Autodesk Inventor part; units mm, degrees
(part 2 of 7)
  arc A582 (128.3559, 101.1967) -> (128.4338, 100.8049) centre (148.5, 105) ccw
  arc A583 (128.7164, 99.628) -> (128.8248, 99.2435) centre (148.5, 105) ccw
  arc A584 (129.1989, 98.0923) -> (129.3371, 97.7175) centre (148.5, 105) ccw
  arc A585 (129.8003, 96.5993) -> (129.9676, 96.2365) centre (148.5, 105) ccw
  arc A586 (130.5171, 95.158) -> (130.7123, 94.8095) centre (148.5, 105) ccw
  arc A587 (131.3447, 93.7774) -> (131.5666, 93.4453) centre (148.5, 105) ccw
  arc A588 (132.2781, 92.466) -> (132.5254, 92.1523) centre (148.5, 105) ccw
  arc A589 (133.3115, 91.2319) -> (133.5827, 90.9386) centre (148.5, 105) ccw
  arc A590 (134.4386, 90.0827) -> (134.7319, 89.8115) centre (148.5, 105) ccw
  arc A591 (135.6523, 89.0254) -> (135.966, 88.7781) centre (148.5, 105) ccw
  arc A592 (136.9453, 88.0666) -> (137.2774, 87.8447) centre (148.5, 105) ccw
  arc A593 (138.3095, 87.2123) -> (138.658, 87.0171) centre (148.5, 105) ccw
  arc A594 (139.7365, 86.4676) -> (140.0993, 86.3003) centre (148.5, 105) ccw
  arc A595 (141.2175, 85.8371) -> (141.5923, 85.6989) centre (148.5, 105) ccw
  arc A596 (142.7435, 85.3248) -> (143.128, 85.2164) centre (148.5, 105) ccw
  arc A597 (144.3049, 84.9338) -> (144.6967, 84.8559) centre (148.5, 105) ccw
  arc A598 (145.8922, 84.6665) -> (146.2889, 84.6196) centre (148.5, 105) ccw
  arc A599 (147.4956, 84.5246) -> (147.8948, 84.5089) centre (148.5, 105) ccw
  arc A600 (149.1052, 84.5089) -> (149.5044, 84.5246) centre (148.5, 105) ccw
  arc A601 (150.7111, 84.6196) -> (151.1078, 84.6665) centre (148.5, 105) ccw
  arc A602 (152.3033, 84.8559) -> (152.6951, 84.9338) centre (148.5, 105) ccw
  arc A603 (153.872, 85.2164) -> (154.2565, 85.3248) centre (148.5, 105) ccw
  arc A604 (155.4077, 85.6989) -> (155.7825, 85.8371) centre (148.5, 105) ccw
  arc A605 (156.9007, 86.3003) -> (157.2635, 86.4676) centre (148.5, 105) ccw
  arc A606 (158.342, 87.0171) -> (158.6905, 87.2123) centre (148.5, 105) ccw
  arc A607 (159.7226, 87.8447) -> (160.0547, 88.0666) centre (148.5, 105) ccw
  arc A608 (161.034, 88.7781) -> (161.3477, 89.0254) centre (148.5, 105) ccw
  arc A609 (162.2681, 89.8115) -> (162.5614, 90.0827) centre (148.5, 105) ccw
  arc A610 (163.4173, 90.9386) -> (163.6885, 91.2319) centre (148.5, 105) ccw
  arc A611 (164.4746, 92.1523) -> (164.7219, 92.466) centre (148.5, 105) ccw
  arc A612 (165.4334, 93.4453) -> (165.6553, 93.7774) centre (148.5, 105) ccw
  arc A613 (166.2877, 94.8095) -> (166.4829, 95.158) centre (148.5, 105) ccw
  arc A614 (167.0324, 96.2365) -> (167.1997, 96.5993) centre (148.5, 105) ccw
  arc A615 (167.6629, 97.7175) -> (167.8011, 98.0923) centre (148.5, 105) ccw
  arc A616 (168.1752, 99.2435) -> (168.2836, 99.628) centre (148.5, 105) ccw
  arc A617 (168.5662, 100.8049) -> (168.6441, 101.1967) centre (148.5, 105) ccw
  arc A618 (168.8335, 102.3922) -> (168.8804, 102.7889) centre (148.5, 105) ccw
  arc A619 (168.9754, 103.9956) -> (168.9911, 104.3948) centre (148.5, 105) ccw
  arc A620 (168.9911, 105.6052) -> (168.9754, 106.0044) centre (148.5, 105) ccw
  arc A621 (168.8804, 107.2111) -> (168.8335, 107.6078) centre (148.5, 105) ccw
  arc A622 (168.6441, 108.8033) -> (168.5662, 109.1951) centre (148.5, 105) ccw
  arc A623 (168.2836, 110.372) -> (168.1752, 110.7565) centre (148.5, 105) ccw
  arc A624 (167.8011, 111.9077) -> (167.6629, 112.2825) centre (148.5, 105) ccw
  arc A625 (167.1997, 113.4007) -> (167.0324, 113.7635) centre (148.5, 105) ccw
  arc A626 (166.4829, 114.842) -> (166.2877, 115.1905) centre (148.5, 105) ccw
  arc A627 (165.6553, 116.2226) -> (165.4334, 116.5547) centre (148.5, 105) ccw
  arc A628 (164.7219, 117.534) -> (164.4746, 117.8477) centre (148.5, 105) ccw
  arc A629 (163.6885, 118.7681) -> (163.4173, 119.0614) centre (148.5, 105) ccw
  arc A630 (162.5614, 119.9173) -> (162.2681, 120.1885) centre (148.5, 105) ccw
  arc A631 (161.3477, 120.9746) -> (161.034, 121.2219) centre (148.5, 105) ccw
  arc A632 (160.0547, 121.9334) -> (159.7226, 122.1553) centre (148.5, 105) ccw
  arc A633 (158.6905, 122.7877) -> (158.342, 122.9829) centre (148.5, 105) ccw
  arc A634 (157.2635, 123.5324) -> (156.9007, 123.6997) centre (148.5, 105) ccw
  arc A635 (155.7825, 124.1629) -> (155.4077, 124.3011) centre (148.5, 105) ccw
  arc A636 (154.2565, 124.6752) -> (153.872, 124.7836) centre (148.5, 105) ccw
  arc A637 (152.6951, 125.0662) -> (152.3033, 125.1441) centre (148.5, 105) ccw
  arc A638 (151.1078, 125.3335) -> (150.7111, 125.3804) centre (148.5, 105) ccw
  arc A639 (149.5044, 125.4754) -> (149.1052, 125.4911) centre (148.5, 105) ccw
  line L0 (126, 105) -> (171, 105)
  line L1 (148.5, 82.5) -> (148.5, 127.5)
  line L2 (189, 125.5) -> (259, 125.5)
  line L3 (189, 117.5) -> (259, 117.5)
  line L4 (189, 109.5) -> (259, 109.5)
  line L5 (189, 101.5) -> (259, 101.5)
  line L6 (189, 93.5) -> (259, 93.5)
  line L7 (189, 85.5) -> (259, 85.5)
  line L8 (189, 77.5) -> (259, 77.5)
  line L9 (189, 69.5) -> (259, 69.5)
  line L10 (189, 61.5) -> (259, 61.5)
  line L11 (189, 53.5) -> (259, 53.5)
  line L12 (189, 45.5) -> (259, 45.5)
  line L13 (189, 37.5) -> (259, 37.5)
  line L14 (189, 29.5) -> (259, 29.5)
  line L15 (189, 125.5) -> (189, 29.5)
  line L16 (259, 125.5) -> (259, 29.5)
  line L17 (224, 117.5) -> (224, 29.5)
  arc A640 (149.1982, 109.7586) -> (149.1615, 109.6213) centre (149.7545, 109.5365) ccw
  arc A641 (149.402, 110.1264) -> (149.1982, 109.7586) centre (150.7515, 109.1382) ccw
  arc A642 (150.0725, 110.7903) -> (149.402, 110.1264) centre (151.8157, 108.3591) ccw
  arc A643 (146.2672, 109.2599) -> (146.3182, 109.1272) centre (146.8478, 109.4071) ccw
  arc A644 (146.2159, 109.6791) -> (146.2672, 109.2599) centre (147.8885, 109.671) ccw
  arc A645 (146.3688, 110.6087) -> (146.2159, 109.6791) centre (149.2074, 109.6645) ccw
  arc A646 (144.1897, 107.1339) -> (144.309, 107.0566) centre (144.5729, 107.5943) ccw
  arc A647 (143.9018, 107.4429) -> (144.1897, 107.1339) centre (145.2598, 108.4195) ccw
  arc A648 (143.4791, 108.2848) -> (143.9018, 107.4429) centre (146.3305, 109.1895) ccw
  arc A649 (143.7586, 104.1928) -> (143.9006, 104.2004) centre (143.7981, 104.7905) ccw
  arc A650 (143.3441, 104.2736) -> (143.7586, 104.1928) centre (143.8687, 105.8619) ccw
  arc A651 (142.5072, 104.7063) -> (143.3441, 104.2736) centre (144.2823, 107.1142) ccw
  arc A652 (145.1386, 101.5601) -> (145.249, 101.6496) centre (144.8192, 102.0668) ccw
  arc A653 (144.7558, 101.3818) -> (145.1386, 101.5601) centre (144.2466, 102.9751) ccw
  arc A654 (143.8244, 101.2399) -> (144.7558, 101.3818) centre (143.8452, 104.2313) ccw
  arc A655 (147.8018, 100.2415) -> (147.8385, 100.3788) centre (147.2456, 100.4636) ccw
  arc A656 (147.5969, 99.8722) -> (147.8018, 100.2415) centre (146.2485, 100.8619) ccw
  arc A657 (146.9268, 99.2099) -> (147.5969, 99.8722) centre (145.1853, 101.6423) ccw
  arc A658 (150.7315, 100.7396) -> (150.6805, 100.8723) centre (150.1509, 100.5924) ccw
  arc A659 (150.7828, 100.3204) -> (150.7315, 100.7396) centre (149.1102, 100.3285) ccw
  arc A660 (150.6299, 99.3908) -> (150.7828, 100.3204) centre (147.7913, 100.335) ccw
  arc A661 (152.8095, 102.8649) -> (152.6903, 102.9423) centre (152.4263, 102.4046) ccw
  arc A662 (153.0974, 102.5559) -> (152.8095, 102.8649) centre (151.7394, 101.5794) ccw
  arc A663 (153.5202, 101.714) -> (153.0974, 102.5559) centre (150.6687, 100.8093) ccw
  arc A664 (153.2414, 105.8058) -> (153.0995, 105.7982) centre (153.202, 105.2081) ccw
  arc A665 (153.656, 105.725) -> (153.2414, 105.8058) centre (153.1314, 104.1367) ccw
  arc A666 (154.4929, 105.2923) -> (153.656, 105.725) centre (152.7177, 102.8844) ccw
  arc A667 (151.8623, 108.4388) -> (151.7519, 108.3493) centre (152.1817, 107.9321) ccw
  arc A668 (152.2451, 108.6171) -> (151.8623, 108.4388) centre (152.7543, 107.0239) ccw
  arc A669 (153.1765, 108.759) -> (152.2451, 108.6171) centre (153.1557, 105.7676) ccw
  arc A670 (147.8392, 109.6213) -> (147.8025, 109.7587) centre (147.2462, 109.5365) ccw
  arc A671 (147.8025, 109.7587) -> (147.5976, 110.128) centre (146.2492, 109.1383) ccw
  arc A672 (147.5976, 110.128) -> (146.9275, 110.7903) centre (145.186, 108.3579) ccw
  arc A673 (145.2491, 108.3503) -> (145.1386, 108.4399) centre (144.8192, 107.9332) ccw
  arc A674 (145.1386, 108.4399) -> (144.7558, 108.6182) centre (144.2466, 107.0249) ccw
  arc A675 (144.7558, 108.6182) -> (143.8244, 108.7601) centre (143.8452, 105.7687) ccw
  arc A676 (143.9007, 105.7996) -> (143.7586, 105.8072) centre (143.7981, 105.2095) ccw
  arc A677 (143.7586, 105.8072) -> (143.3441, 105.7264) centre (143.8687, 104.1381) ccw
  arc A678 (143.3441, 105.7264) -> (142.5072, 105.2937) centre (144.2823, 102.8858) ccw
  arc A679 (144.309, 102.9435) -> (144.1897, 102.8661) centre (144.5729, 102.4057) ccw
  arc A680 (144.1897, 102.8661) -> (143.9018, 102.5571) centre (145.2598, 101.5805) ccw
  arc A681 (143.9018, 102.5571) -> (143.4791, 101.7152) centre (146.3305, 100.8105) ccw
  arc A682 (146.3189, 100.8726) -> (146.2679, 100.7399) centre (146.8485, 100.5927) ccw
  arc A683 (146.2679, 100.7399) -> (146.2166, 100.3207) centre (147.8892, 100.3288) ccw
  arc A684 (146.2166, 100.3207) -> (146.3695, 99.391) centre (149.2081, 100.3352) ccw
  arc A685 (149.1608, 100.3787) -> (149.1975, 100.2413) centre (149.7538, 100.4635) ccw
  arc A686 (149.1975, 100.2413) -> (149.4024, 99.872) centre (150.7508, 100.8617) ccw
  arc A687 (149.4024, 99.872) -> (150.0725, 99.2097) centre (151.814, 101.6421) ccw
  arc A688 (151.7509, 101.6497) -> (151.8614, 101.5601) centre (152.1808, 102.0668) ccw
  arc A689 (151.8614, 101.5601) -> (152.2442, 101.3818) centre (152.7534, 102.9751) ccw
  arc A690 (152.2442, 101.3818) -> (153.1756, 101.2399) centre (153.1548, 104.2313) ccw
  arc A691 (153.0993, 104.2004) -> (153.2414, 104.1928) centre (153.2019, 104.7905) ccw
  arc A692 (153.2414, 104.1928) -> (153.6559, 104.2736) centre (153.1313, 105.8619) ccw
  arc A693 (153.6559, 104.2736) -> (154.4928, 104.7063) centre (152.7177, 107.1142) ccw
  arc A694 (152.691, 107.0565) -> (152.8103, 107.1339) centre (152.4271, 107.5943) ccw
  arc A695 (152.8103, 107.1339) -> (153.0982, 107.4429) centre (151.7402, 108.4195) ccw
  arc A696 (153.0982, 107.4429) -> (153.5209, 108.2848) centre (150.6695, 109.1895) ccw
  arc A697 (150.6818, 109.1272) -> (150.7328, 109.2599) centre (150.1522, 109.4071) ccw
  arc A698 (150.7328, 109.2599) -> (150.7841, 109.6791) centre (149.1115, 109.671) ccw
  arc A699 (150.7841, 109.6791) -> (150.6312, 110.6087) centre (147.7926, 109.6645) ccw
  arc A700 (149.0314, 108.7125) -> (147.9691, 108.7126) centre (148.5, 105) ccw
  arc A701 (146.7471, 108.3155) -> (145.8883, 107.6915) centre (148.5, 105) ccw
  arc A702 (145.1331, 106.652) -> (144.8051, 105.6424) centre (148.5, 105) ccw
  arc A703 (144.8051, 104.3575) -> (145.1332, 103.3479) centre (148.5, 105) ccw
  arc A704 (145.8884, 102.3084) -> (146.7478, 101.6841) centre (148.5, 105) ccw
  arc A705 (147.9686, 101.2875) -> (149.0308, 101.2874) centre (148.5, 105) ccw
  arc A706 (150.2516, 101.6838) -> (151.1117, 102.3085) centre (148.5, 105) ccw
  arc A707 (151.8663, 103.3467) -> (152.1949, 104.3576) centre (148.5, 105) ccw
  arc A708 (152.1951, 105.6411) -> (151.8668, 106.6521) centre (148.5, 105) ccw
  arc A709 (151.1126, 107.6906) -> (150.2528, 108.3155) centre (148.5, 105) ccw
  arc A710 (146.9275, 110.7903) -> (146.3688, 110.6087) centre (148.5, 105) ccw
  arc A711 (143.8244, 108.7601) -> (143.4791, 108.2848) centre (148.5, 105) ccw
  arc A712 (142.5072, 105.2937) -> (142.5072, 104.7063) centre (148.5, 105) ccw
  arc A713 (143.4791, 101.7152) -> (143.8244, 101.2399) centre (148.5, 105) ccw
  arc A714 (146.3695, 99.391) -> (146.9268, 99.2099) centre (148.5, 105) ccw
  arc A715 (150.0725, 99.2097) -> (150.6299, 99.3908) centre (148.5, 105) ccw
  arc A716 (153.1756, 101.2399) -> (153.5202, 101.714) centre (148.5, 105) ccw
  arc A717 (154.4928, 104.7063) -> (154.4929, 105.2923) centre (148.5, 105) ccw
  arc A718 (153.5209, 108.2848) -> (153.1765, 108.759) centre (148.5, 105) ccw
  arc A719 (150.6312, 110.6087) -> (150.0725, 110.7903) centre (148.5, 105) ccw
  line L18 (149.0314, 108.7125) -> (149.1615, 109.6213)
  line L19 (146.7471, 108.3155) -> (146.3182, 109.1272)
  line L20 (145.1331, 106.652) -> (144.309, 107.0566)
  line L21 (144.8051, 104.3575) -> (143.9006, 104.2004)
  line L22 (145.8884, 102.3084) -> (145.249, 101.6496)
  line L23 (147.9686, 101.2875) -> (147.8385, 100.3788)
  line L24 (150.2516, 101.6838) -> (150.6805, 100.8723)
  line L25 (151.8663, 103.3467) -> (152.6903, 102.9423)
  line L26 (152.1951, 105.6411) -> (153.0995, 105.7982)
  line L27 (151.1126, 107.6906) -> (151.7519, 108.3493)
  line L28 (147.9691, 108.7126) -> (147.8392, 109.6213)
  line L29 (145.8883, 107.6915) -> (145.2491, 108.3503)
  line L30 (144.8051, 105.6424) -> (143.9007, 105.7996)
  line L31 (145.1332, 103.3479) -> (144.309, 102.9435)
  line L32 (146.7478, 101.6841) -> (146.3189, 100.8726)
  line L33 (149.0308, 101.2874) -> (149.1608, 100.3787)
  line L34 (151.1117, 102.3085) -> (151.7509, 101.6497)
  line L35 (152.1949, 104.3576) -> (153.0993, 104.2004)
  line L36 (151.8668, 106.6521) -> (152.691, 107.0565)
  line L37 (150.2528, 108.3155) -> (150.6818, 109.1272)
  line L38 (140.5, 105) -> (156.5, 105)
  line L39 (148.5, 97) -> (148.5, 113)
  line L40 (174.5, 111) -> (244.5, 111)
  line L41 (174.5, 103) -> (244.5, 103)
  line L42 (174.5, 95) -> (244.5, 95)
  line L43 (174.5, 87) -> (244.5, 87)
  line L44 (174.5, 79) -> (244.5, 79)
  line L45 (174.5, 71) -> (244.5, 71)
  line L46 (174.5, 63) -> (244.5, 63)
  line L47 (174.5, 55) -> (244.5, 55)
  line L48 (174.5, 47) -> (244.5, 47)
  line L49 (174.5, 39) -> (244.5, 39)
  line L50 (174.5, 31) -> (244.5, 31)
  line L51 (174.5, 23) -> (244.5, 23)
  line L52 (174.5, 15) -> (244.5, 15)
  line L53 (174.5, 111) -> (174.5, 15)
  line L54 (244.5, 111) -> (244.5, 15)
  line L55 (209.5, 103) -> (209.5, 15)
  point P0 (0, 0)
  point P1 (195, 119.5)
  point P2 (197.5, 111.5)
  point P3 (197.5, 103.5)
  point P4 (195, 95.5)
  point P5 (197.5, 87.5)
  point P6 (192.5, 79.5)
  point P7 (195, 71.5)
  point P8 (195, 63.5)
  point P9 (195, 55.5)
  point P10 (197.5, 47.5)
  point P11 (197.5, 39.5)
  point P12 (195, 31.5)
  point P13 (225, 111.5)
  point P14 (240, 103.5)
  point P15 (238.75, 95.5)
  point P16 (237.5, 87.5)
  point P17 (240, 79.5)
  point P18 (233.75, 71.5)
  point P19 (240, 63.5)
  point P20 (236.25, 55.5)
  point P21 (235, 47.5)
  point P22 (242.5, 39.5)
  point P23 (242.5, 31.5)
  point P24 (149.5, 141)
  point P25 (149.5, 135)
  point P26 (165.6875, 141)
  point P27 (167.8125, 135)
  point P28 (180.5, 105)
  point P29 (183, 97)
  point P30 (183, 89)
  point P31 (180.5, 81)
  point P32 (183, 73)
  point P33 (178, 65)
  point P34 (180.5, 57)
  point P35 (180.5, 49)
  point P36 (180.5, 41)
  point P37 (183, 33)
  point P38 (183, 25)
  point P39 (180.5, 17)
  point P40 (210.5, 97)
  point P41 (225.5, 89)
  point P42 (226.75, 81)
  point P43 (223, 73)
  point P44 (225.5, 65)
  point P45 (220.5, 57)
  point P46 (225.5, 49)
  point P47 (224.25, 41)
  point P48 (220.5, 33)
  point P49 (228, 25)
  point P50 (228, 17)
  point P51 (149.5, 126.5)
  point P52 (149.5, 120.5)
  point P53 (167.8125, 126.5)
  point P54 (168.875, 120.5)
  constraints: 1120 point on circle, 560 centre point, 534 equal radius, 410 tangent, 104 end point, 84 horizontal, 26 parallel, 9 concentric, 4 midpoint, 4 perpendicular, 2 horizontal alignment, 2 vertical alignment, 586 other
extrude "押し出し1" add sketch "スケッチ1" along normal blind 3 contours A1 A2 A639 A479 A478 A477 A559 A237 A238 A239 A638 A476 A475 A474 A558 A234 A235 A236 A637 A473 A472 A471 A557 A231 A232 A233 A636 A470 A469 A468 A556 A228 A229 A230 A635 A467 A466 A465 A555 A225 A226 A227 A634 A464 A463 A462 A554 A222 A223 A224 A633 A461 A460 A459 A553 A219 A220 A221 A632 A458 A457 A456 A552 A216 A217 A218 A631 A455 A454 A453 A551 A213 A214 A215 A630 A452 A451 A450 A550 A210 A211 A212 A629 A449 A448 A447 A549 A207 A208 A209 A628 A446 A445 A444 A548 A204 A205 A206 A627 A443 A442 A441 A547 A201 A202 A203 A626 A440 A439 A438 A546 A198 A199 A200 A625 A437 A436 A435 A545 A195 A196 A197 A624 A434 A433 A432 A544 A192 A193 A194 A623 A431 A430 A429 A543 A189 A190 A191 A622 A428 A427 A426 A542 A186 A187 A188 A621 A425 A424 A423 A541 A183 A184 A185 A620 A422 A421 A420 A540 L0 A717 A666 A665 A664 L26 A708 L36 A694 A695 A696 A718 A669 A668 A667 L27 A709 L37 A697 A698 A699 A719 A642 A641 A640 L18 A700 L1 A480 A0 | L1 A700 L28 A670 A671 A672 A710 A645 A644 A643 L19 A701 L29 A673 A674 A675 A711 A648 A647 A646 L20 A702 L30 A676 A677 A678 A712 L0 A500 A60 A61 A62 A579 A299 A298 A297 A499 A57 A58 A59 A578 A296 A295 A294 A498 A54 A55 A56 A577 A293 A292 A291 A497 A51 A52 A53 A576 A290 A289 A288 A496 A48 A49 A50 A575 A287 A286 A285 A495 A45 A46 A47 A574 A284 A283 A282 A494 A42 A43 A44 A573 A281 A280 A279 A493 A39 A40 A41 A572 A278 A277 A276 A492 A36 A37 A38 A571 A275 A274 A273 A491 A33 A34 A35 A570 A272 A271 A270 A490 A30 A31 A32 A569 A269 A268 A267 A489 A27 A28 A29 A568 A266 A265 A264 A488 A24 A25 A26 A567 A263 A262 A261 A487 A21 A22 A23 A566 A260 A259 A258 A486 A18 A19 A20 A565 A257 A256 A255 A485 A15 A16 A17 A564 A254 A253 A252 A484 A12 A13 A14 A563 A251 A250 A249 A483 A9 A10 A11 A562 A248 A247 A246 A482 A6 A7 A8 A561 A245 A244 A243 A481 A3 A4 A5 A560 A242 A241 A240 A480 | A700 L18 A640 A641 A642 A719 A699 A698 A697 L37 A709 L27 A667 A668 A669 A718 A696 A695 A694 L36 A708 L26 A664 A665 A666 A717 L0 L1 | L1 L0 A712 A678 A677 A676 L30 A702 L20 A646 A647 A648 A711 A675 A674 A673 L29 A701 L19 A643 A644 A645 A710 A672 A671 A670 L28 A700 | L1 A705 L23 A655 A656 A657 A714 A684 A683 A682 L32 A704 L22 A652 A653 A654 A713 A681 A680 A679 L31 A703 L21 A649 A650 A651 A712 L0 | L0 A717 A693 A692 A691 L35 A707 L25 A661 A662 A663 A716 A690 A689 A688 L34 A706 L24 A658 A659 A660 A715 A687 A686 A685 L33 A705 L1 | A712 A651 A650 A649 L21 A703 L31 A679 A680 A681 A713 A654 A653 A652 L22 A704 L32 A682 A683 A684 A714 A657 A656 A655 L23 A705 L1 A520 A120 A121 A122 A599 A359 A358 A357 A519 A117 A118 A119 A598 A356 A355 A354 A518 A114 A115 A116 A597 A353 A352 A351 A517 A111 A112 A113 A596 A350 A349 A348 A516 A108 A109 A110 A595 A347 A346 A345 A515 A105 A106 A107 A594 A344 A343 A342 A514 A102 A103 A104 A593 A341 A340 A339 A513 A99 A100 A101 A592 A338 A337 A336 A512 A96 A97 A98 A591 A335 A334 A333 A511 A93 A94 A95 A590 A332 A331 A330 A510 A90 A91 A92 A589 A329 A328 A327 A509 A87 A88 A89 A588 A326 A325 A324 A508 A84 A85 A86 A587 A323 A322 A321 A507 A81 A82 A83 A586 A320 A319 A318 A506 A78 A79 A80 A585 A317 A316 A315 A505 A75 A76 A77 A584 A314 A313 A312 A504 A72 A73 A74 A583 A311 A310 A309 A503 A69 A70 A71 A582 A308 A307 A306 A502 A66 A67 A68 A581 A305 A304 A303 A501 A63 A64 A65 A580 A302 A301 A300 A500 L0 | L0 A540 A180 A181 A182 A619 A419 A418 A417 A539 A177 A178 A179 A618 A416 A415 A414 A538 A174 A175 A176 A617 A413 A412 A411 A537 A171 A172 A173 A616 A410 A409 A408 A536 A168 A169 A170 A615 A407 A406 A405 A535 A165 A166 A167 A614 A404 A403 A402 A534 A162 A163 A164 A613 A401 A400 A399 A533 A159 A160 A161 A612 A398 A397 A396 A532 A156 A157 A158 A611 A395 A394 A393 A531 A153 A154 A155 A610 A392 A391 A390 A530 A150 A151 A152 A609 A389 A388 A387 A529 A147 A148 A149 A608 A386 A385 A384 A528 A144 A145 A146 A607 A383 A382 A381 A527 A141 A142 A143 A606 A380 A379 A378 A526 A138 A139 A140 A605 A377 A376 A375 A525 A135 A136 A137 A604 A374 A373 A372 A524 A132 A133 A134 A603 A371 A370 A369 A523 A129 A130 A131 A602 A368 A367 A366 A522 A126 A127 A128 A601 A365 A364 A363 A521 A123 A124 A125 A600 A362 A361 A360 A520 L1 A705 L33 A685 A686 A687 A715 A660 A659 A658 L24 A706 L34 A688 A689 A690 A716 A663 A662 A661 L25 A707 L35 A691 A692 A693 A717
sketch "スケッチ3" plane through (0, 0, 0) normal (0, 0, -1) x (-1, 0, 0)
  arc A0 (-148.7771, 124.6719) -> (-148.9109, 125.0429) centre (-154.869, 122.6849) ccw projected
  arc A1 (-148.6896, 124.3741) -> (-148.7771, 124.6719) centre (-153.7892, 123.0371) ccw projected
  arc A2 (-148.3104, 124.3741) -> (-148.6896, 124.3741) centre (-148.5, 105) ccw projected
  arc A3 (-148.2229, 124.6719) -> (-148.3104, 124.3741) centre (-143.2108, 123.0371) ccw projected
  arc A4 (-148.0891, 125.0429) -> (-148.2229, 124.6719) centre (-142.131, 122.6849) ccw projected
  arc A5 (-147.8948, 125.4911) -> (-148.0891, 125.0429) centre (-141.0342, 122.2508) ccw projected
  arc A6 (-147.4956, 125.4754) -> (-147.8948, 125.4911) centre (-148.5, 105) ccw projected
  arc A7 (-147.3371, 125.0133) -> (-147.4956, 125.4754) centre (-154.5894, 122.7834) ccw projected
  arc A8 (-147.2329, 124.633) -> (-147.3371, 125.0133) centre (-153.4618, 123.1301) ccw projected
  arc A9 (-147.169, 124.3292) -> (-147.2329, 124.633) centre (-152.3577, 123.3965) ccw projected
  arc A10 (-146.7909, 124.2995) -> (-147.169, 124.3292) centre (-148.5, 105) ccw projected
  arc A11 (-146.6803, 124.5895) -> (-146.7909, 124.2995) centre (-141.8119, 122.5665) ccw projected
  arc A12 (-146.5178, 124.9489) -> (-146.6803, 124.5895) centre (-140.7631, 122.1307) ccw projected
  arc A13 (-146.2889, 125.3804) -> (-146.5178, 124.9489) centre (-139.7037, 121.6119) ccw projected
  arc A14 (-145.8922, 125.3335) -> (-146.2889, 125.3804) centre (-148.5, 105) ccw projected
  arc A15 (-145.7705, 124.8604) -> (-145.8922, 125.3335) centre (-153.1753, 123.2064) ccw projected
  arc A16 (-145.6964, 124.473) -> (-145.7705, 124.8604) centre (-152.0241, 123.4635) ccw projected
  arc A17 (-145.6565, 124.1652) -> (-145.6964, 124.473) centre (-150.9025, 123.6425) ccw projected
  arc A18 (-145.2819, 124.1059) -> (-145.6565, 124.1652) centre (-148.5, 105) ccw projected
  arc A19 (-145.1489, 124.3863) -> (-145.2819, 124.1059) centre (-140.4543, 121.9876) ccw projected
  arc A20 (-144.9587, 124.7318) -> (-145.1489, 124.3863) centre (-139.4429, 121.4708) ccw projected
  arc A21 (-144.6967, 125.1441) -> (-144.9587, 124.7318) centre (-138.4274, 120.8705) ccw projected
  arc A22 (-144.3049, 125.0662) -> (-144.6967, 125.1441) centre (-148.5, 105) ccw projected
  arc A23 (-144.2207, 124.585) -> (-144.3049, 125.0662) centre (-151.7324, 123.517) ccw projected
  arc A24 (-144.1772, 124.193) -> (-144.2207, 124.585) centre (-150.5646, 123.6831) ccw projected
  arc A25 (-144.1616, 123.883) -> (-144.1772, 124.193) centre (-149.4324, 123.7735) ccw projected
  arc A26 (-143.7928, 123.7945) -> (-144.1616, 123.883) centre (-148.5, 105) ccw projected
  arc A27 (-143.6382, 124.0636) -> (-143.7928, 123.7945) centre (-139.1463, 121.304) ccw projected
  arc A28 (-143.4215, 124.3932) -> (-143.6382, 124.0636) centre (-138.1785, 120.7095) ccw projected
  arc A29 (-143.128, 124.7836) -> (-143.4215, 124.3932) centre (-137.2133, 120.0313) ccw projected
  arc A30 (-142.7435, 124.6752) -> (-143.128, 124.7836) centre (-148.5, 105) ccw projected
  arc A31 (-142.6972, 124.1889) -> (-142.7435, 124.6752) centre (-150.2696, 123.7136) ccw projected
  arc A32 (-142.6846, 123.7947) -> (-142.6972, 124.1889) centre (-149.0924, 123.7875) ccw projected
  arc A33 (-142.6934, 123.4844) -> (-142.6846, 123.7947) centre (-147.9566, 123.7888) ccw projected
  arc A34 (-142.3327, 123.3672) -> (-142.6934, 123.4844) centre (-148.5, 105) ccw projected
  arc A35 (-142.1575, 123.6234) -> (-142.3327, 123.3672) centre (-137.8959, 120.5199) ccw projected
  arc A36 (-141.9156, 123.9349) -> (-142.1575, 123.6234) centre (-136.9778, 119.8512) ccw projected
  arc A37 (-141.5923, 124.3011) -> (-141.9156, 123.9349) centre (-136.0688, 119.0994) ccw projected
  arc A38 (-141.2175, 124.1629) -> (-141.5923, 124.3011) centre (-148.5, 105) ccw projected
  arc A39 (-141.2096, 123.6745) -> (-141.2175, 124.1629) centre (-148.7959, 123.7947) ccw projected
  arc A40 (-141.228, 123.2805) -> (-141.2096, 123.6745) centre (-147.6165, 123.776) ccw projected
  arc A41 (-141.2611, 122.9719) -> (-141.228, 123.2805) centre (-146.4841, 123.6882) ccw projected
  arc A42 (-140.9107, 122.8267) -> (-141.2611, 122.9719) centre (-148.5, 105) ccw projected
  arc A43 (-140.7158, 123.0684) -> (-140.9107, 122.8267) centre (-136.7109, 119.64) ccw projected
  arc A44 (-140.4503, 123.36) -> (-140.7158, 123.0684) centre (-135.8481, 118.9014) ccw projected
  arc A45 (-140.0993, 123.6997) -> (-140.4503, 123.36) centre (-135.0009, 118.0806) ccw projected
  arc A46 (-139.7365, 123.5324) -> (-140.0993, 123.6997) centre (-148.5, 105) ccw projected
  arc A47 (-139.7669, 123.0449) -> (-139.7365, 123.5324) centre (-147.3204, 123.76) ccw projected
  arc A48 (-139.8161, 122.6536) -> (-139.7669, 123.0449) centre (-146.1461, 123.6488) ccw projected
  arc A49 (-139.8733, 122.3485) -> (-139.8161, 122.6536) centre (-145.024, 123.4724) ccw projected
  arc A50 (-139.5354, 122.1763) -> (-139.8733, 122.3485) centre (-148.5, 105) ccw projected
  arc A51 (-139.3222, 122.4019) -> (-139.5354, 122.1763) centre (-135.5986, 118.6699) ccw projected
  arc A52 (-139.0346, 122.6718) -> (-139.3222, 122.4019) centre (-134.7964, 117.8659) ccw projected
  arc A53 (-138.658, 122.9829) -> (-139.0346, 122.6718) centre (-134.0162, 116.9812) ccw projected
  arc A54 (-138.3095, 122.7877) -> (-138.658, 122.9829) centre (-148.5, 105) ccw projected
  arc A55 (-138.378, 122.3041) -> (-138.3095, 122.7877) centre (-145.8522, 123.6096) ccw projected
  arc A56 (-138.4578, 121.9178) -> (-138.378, 122.3041) centre (-144.6901, 123.4067) ccw projected
  arc A57 (-138.5388, 121.6182) -> (-138.4578, 121.9178) centre (-143.5854, 123.1428) ccw projected
  arc A58 (-138.2154, 121.42) -> (-138.5388, 121.6182) centre (-148.5, 105) ccw projected
  arc A59 (-137.9852, 121.6282) -> (-138.2154, 121.42) centre (-134.5659, 117.6156) ccw projected
  arc A60 (-137.6773, 121.8747) -> (-137.9852, 121.6282) centre (-133.8292, 116.7511) ccw projected
  arc A61 (-137.2774, 122.1553) -> (-137.6773, 121.8747) centre (-133.1208, 115.8078) ccw projected
  arc A62 (-136.9453, 121.9334) -> (-137.2774, 122.1553) centre (-148.5, 105) ccw projected
  arc A63 (-137.0515, 121.4566) -> (-136.9453, 121.9334) centre (-144.4002, 123.3445) ccw projected
  arc A64 (-137.1614, 121.0778) -> (-137.0515, 121.4566) centre (-143.2577, 123.051) ccw projected
  arc A65 (-137.2656, 120.7854) -> (-137.1614, 121.0778) centre (-142.1771, 122.7012) ccw projected
  arc A66 (-136.9588, 120.5625) -> (-137.2656, 120.7854) centre (-148.5, 105) ccw projected
  arc A67 (-136.7129, 120.752) -> (-136.9588, 120.5625) centre (-133.619, 116.4834) ccw projected
  arc A68 (-136.3866, 120.9735) -> (-136.7129, 120.752) centre (-132.9524, 115.5638) ccw projected
  arc A69 (-135.966, 121.2219) -> (-136.3866, 120.9735) centre (-132.3202, 114.5679) ccw projected
  arc A70 (-135.6523, 120.9746) -> (-135.966, 121.2219) centre (-148.5, 105) ccw projected
  arc A71 (-135.7957, 120.5076) -> (-135.6523, 120.9746) centre (-142.9736, 122.9663) ccw projected
  arc A72 (-135.9349, 120.1386) -> (-135.7957, 120.5076) centre (-141.8576, 122.5841) ccw projected
  arc A73 (-136.0617, 119.8553) -> (-135.9349, 120.1386) centre (-140.8078, 122.1506) ccw projected
  arc A74 (-135.7734, 119.609) -> (-136.0617, 119.8553) centre (-148.5, 105) ccw projected
  arc A75 (-135.5134, 119.7786) -> (-135.7734, 119.609) centre (-132.7639, 115.2805) ccw projected
  arc A76 (-135.1707, 119.9739) -> (-135.5134, 119.7786) centre (-132.1715, 114.3114) ccw projected
  arc A77 (-134.7319, 120.1885) -> (-135.1707, 119.9739) centre (-131.6194, 113.2689) ccw projected
  arc A78 (-134.4386, 119.9173) -> (-134.7319, 120.1885) centre (-148.5, 105) ccw projected
  arc A79 (-134.6181, 119.463) -> (-134.4386, 119.9173) centre (-141.581, 122.4773) ccw projected
  arc A80 (-134.7859, 119.1061) -> (-134.6181, 119.463) centre (-140.4985, 122.0087) ccw projected
  arc A81 (-134.9345, 118.8336) -> (-134.7859, 119.1061) centre (-139.4859, 121.4942) ccw projected
  arc A82 (-134.6664, 118.5655) -> (-134.9345, 118.8336) centre (-148.5, 105) ccw projected
  arc A83 (-134.3939, 118.7141) -> (-134.6664, 118.5655) centre (-132.0058, 114.0141) ccw projected
  arc A84 (-134.037, 118.8819) -> (-134.3939, 118.7141) centre (-131.4913, 113.0015) ccw projected
  arc A85 (-133.5827, 119.0614) -> (-134.037, 118.8819) centre (-131.0227, 111.919) ccw projected
  arc A86 (-133.3115, 118.7681) -> (-133.5827, 119.0614) centre (-148.5, 105) ccw projected
  arc A87 (-133.5261, 118.3293) -> (-133.3115, 118.7681) centre (-140.2311, 121.8806) ccw projected
  arc A88 (-133.7214, 117.9866) -> (-133.5261, 118.3293) centre (-139.1886, 121.3285) ccw projected
  arc A89 (-133.891, 117.7266) -> (-133.7214, 117.9866) centre (-138.2195, 120.7361) ccw projected
  arc A90 (-133.6447, 117.4383) -> (-133.891, 117.7266) centre (-148.5, 105) ccw projected
  arc A91 (-133.3614, 117.5651) -> (-133.6447, 117.4383) centre (-131.3494, 112.6922) ccw projected
  arc A92 (-132.9924, 117.7043) -> (-133.3614, 117.5651) centre (-130.9159, 111.6424) ccw projected
  arc A93 (-132.5254, 117.8477) -> (-132.9924, 117.7043) centre (-130.5337, 110.5264) ccw projected
  arc A94 (-132.2781, 117.534) -> (-132.5254, 117.8477) centre (-148.5, 105) ccw projected
  arc A95 (-132.5265, 117.1134) -> (-132.2781, 117.534) centre (-138.9321, 121.1798) ccw projected
  arc A96 (-132.748, 116.7871) -> (-132.5265, 117.1134) centre (-137.9362, 120.5476) ccw projected
  arc A97 (-132.9375, 116.5412) -> (-132.748, 116.7871) centre (-137.0166, 119.881) ccw projected
  arc A98 (-132.7146, 116.2344) -> (-132.9375, 116.5412) centre (-148.5, 105) ccw projected
  arc A99 (-132.4222, 116.3386) -> (-132.7146, 116.2344) centre (-130.7988, 111.3229) ccw projected
  arc A100 (-132.0434, 116.4485) -> (-132.4222, 116.3386) centre (-130.449, 110.2423) ccw projected
  arc A101 (-131.5666, 116.5547) -> (-132.0434, 116.4485) centre (-130.1555, 109.0998) ccw projected
  arc A102 (-131.3447, 116.2226) -> (-131.5666, 116.5547) centre (-148.5, 105) ccw projected
  arc A103 (-131.6253, 115.8227) -> (-131.3447, 116.2226) centre (-137.6922, 120.3792) ccw projected
  arc A104 (-131.8718, 115.5148) -> (-131.6253, 115.8227) centre (-136.7489, 119.6708) ccw projected
  arc A105 (-132.08, 115.2846) -> (-131.8718, 115.5148) centre (-135.8844, 118.9341) ccw projected
  arc A106 (-131.8818, 114.9612) -> (-132.08, 115.2846) centre (-148.5, 105) ccw projected
  arc A107 (-131.5822, 115.0422) -> (-131.8818, 114.9612) centre (-130.3572, 109.9146) ccw projected
  arc A108 (-131.1959, 115.122) -> (-131.5822, 115.0422) centre (-130.0933, 108.8099) ccw projected
  arc A109 (-130.7123, 115.1905) -> (-131.1959, 115.122) centre (-129.8904, 107.6478) ccw projected
  arc A110 (-130.5171, 114.842) -> (-130.7123, 115.1905) centre (-148.5, 105) ccw projected
  arc A111 (-130.8282, 114.4654) -> (-130.5171, 114.842) centre (-136.5188, 119.4838) ccw projected
  arc A112 (-131.0981, 114.1778) -> (-130.8282, 114.4654) centre (-135.6341, 118.7036) ccw projected
  arc A113 (-131.3237, 113.9646) -> (-131.0981, 114.1778) centre (-134.8301, 117.9014) ccw projected
  arc A114 (-131.1515, 113.6267) -> (-131.3237, 113.9646) centre (-148.5, 105) ccw projected
  arc A115 (-130.8464, 113.6839) -> (-131.1515, 113.6267) centre (-130.0276, 108.476) ccw projected
  arc A116 (-130.4551, 113.7331) -> (-130.8464, 113.6839) centre (-129.8512, 107.3539) ccw projected
  arc A117 (-129.9676, 113.7635) -> (-130.4551, 113.7331) centre (-129.74, 106.1796) ccw projected
  arc A118 (-129.8003, 113.4007) -> (-129.9676, 113.7635) centre (-148.5, 105) ccw projected
  arc A119 (-130.14, 113.0497) -> (-129.8003, 113.4007) centre (-135.4194, 118.4991) ccw projected
  arc A120 (-130.4316, 112.7842) -> (-130.14, 113.0497) centre (-134.5986, 117.6519) ccw projected
  arc A121 (-130.6733, 112.5893) -> (-130.4316, 112.7842) centre (-133.86, 116.7891) ccw projected
  arc A122 (-130.5281, 112.2389) -> (-130.6733, 112.5893) centre (-148.5, 105) ccw projected
  arc A123 (-130.2195, 112.272) -> (-130.5281, 112.2389) centre (-129.8118, 107.0159) ccw projected
  arc A124 (-129.8255, 112.2904) -> (-130.2195, 112.272) centre (-129.724, 105.8835) ccw projected
  arc A125 (-129.3371, 112.2825) -> (-129.8255, 112.2904) centre (-129.7053, 104.7041) ccw projected
  arc A126 (-129.1989, 111.9077) -> (-129.3371, 112.2825) centre (-148.5, 105) ccw projected
  arc A127 (-129.5651, 111.5844) -> (-129.1989, 111.9077) centre (-134.4006, 117.4312) ccw projected
  arc A128 (-129.8766, 111.3425) -> (-129.5651, 111.5844) centre (-133.6488, 116.5222) ccw projected
  arc A129 (-130.1328, 111.1673) -> (-129.8766, 111.3425) centre (-132.9801, 115.6041) ccw projected
  arc A130 (-130.0156, 110.8066) -> (-130.1328, 111.1673) centre (-148.5, 105) ccw projected
  arc A131 (-129.7053, 110.8154) -> (-130.0156, 110.8066) centre (-129.7112, 105.5434) ccw projected
  arc A132 (-129.3111, 110.8028) -> (-129.7053, 110.8154) centre (-129.7125, 104.4076) ccw projected
  arc A133 (-128.8248, 110.7565) -> (-129.3111, 110.8028) centre (-129.7864, 103.2304) ccw projected
  arc A134 (-128.7164, 110.372) -> (-128.8248, 110.7565) centre (-148.5, 105) ccw projected
  arc A135 (-129.1068, 110.0785) -> (-128.7164, 110.372) centre (-133.4687, 116.2867) ccw projected
  arc A136 (-129.4364, 109.8618) -> (-129.1068, 110.0785) centre (-132.7905, 115.3215) ccw projected
  arc A137 (-129.7055, 109.7072) -> (-129.4364, 109.8618) centre (-132.196, 114.3537) ccw projected
  arc A138 (-129.617, 109.3384) -> (-129.7055, 109.7072) centre (-148.5, 105) ccw projected
  arc A139 (-129.307, 109.3228) -> (-129.617, 109.3384) centre (-129.7265, 104.0676) ccw projected
  arc A140 (-128.915, 109.2793) -> (-129.307, 109.3228) centre (-129.8169, 102.9354) ccw projected
  arc A141 (-128.4338, 109.1951) -> (-128.915, 109.2793) centre (-129.983, 101.7676) ccw projected
  arc A142 (-128.3559, 108.8033) -> (-128.4338, 109.1951) centre (-148.5, 105) ccw projected
  arc A143 (-128.7682, 108.5413) -> (-128.3559, 108.8033) centre (-132.6295, 115.0726) ccw projected
  arc A144 (-129.1137, 108.3511) -> (-128.7682, 108.5413) centre (-132.0292, 114.0571) ccw projected
  arc A145 (-129.3941, 108.2181) -> (-129.1137, 108.3511) centre (-131.5124, 113.0457) ccw projected
  arc A146 (-129.3348, 107.8435) -> (-129.3941, 108.2181) centre (-148.5, 105) ccw projected
  arc A147 (-129.027, 107.8036) -> (-129.3348, 107.8435) centre (-129.8575, 102.5975) ccw projected
  arc A148 (-128.6396, 107.7295) -> (-129.027, 107.8036) centre (-130.0365, 101.4759) ccw projected
  arc A149 (-128.1665, 107.6078) -> (-128.6396, 107.7295) centre (-130.2936, 100.3247) ccw projected
  arc A150 (-128.1196, 107.2111) -> (-128.1665, 107.6078) centre (-148.5, 105) ccw projected
  arc A151 (-128.5511, 106.9822) -> (-128.1196, 107.2111) centre (-131.8881, 113.7963) ccw projected
  arc A152 (-128.9105, 106.8197) -> (-128.5511, 106.9822) centre (-131.3693, 112.7369) ccw projected
  arc A153 (-129.2005, 106.7091) -> (-128.9105, 106.8197) centre (-130.9335, 111.6881) ccw projected
  arc A154 (-129.1708, 106.331) -> (-129.2005, 106.7091) centre (-148.5, 105) ccw projected
  arc A155 (-128.867, 106.2671) -> (-129.1708, 106.331) centre (-130.1035, 101.1423) ccw projected
  arc A156 (-128.4867, 106.1629) -> (-128.867, 106.2671) centre (-130.3699, 100.0382) ccw projected
  arc A157 (-128.0246, 106.0044) -> (-128.4867, 106.1629) centre (-130.7166, 98.9106) ccw projected
  arc A158 (-128.0089, 105.6052) -> (-128.0246, 106.0044) centre (-148.5, 105) ccw projected
  arc A159 (-128.4571, 105.4109) -> (-128.0089, 105.6052) centre (-131.2492, 112.4658) ccw projected
  arc A160 (-128.8281, 105.2771) -> (-128.4571, 105.4109) centre (-130.8151, 111.369) ccw projected
  arc A161 (-129.1259, 105.1896) -> (-128.8281, 105.2771) centre (-130.4629, 110.2892) ccw projected
  arc A162 (-129.1259, 104.8104) -> (-129.1259, 105.1896) centre (-148.5, 105) ccw projected
  arc A163 (-128.8281, 104.7229) -> (-129.1259, 104.8104) centre (-130.4629, 99.7108) ccw projected
  arc A164 (-128.4571, 104.5891) -> (-128.8281, 104.7229) centre (-130.8151, 98.631) ccw projected
  arc A165 (-128.0089, 104.3948) -> (-128.4571, 104.5891) centre (-131.2492, 97.5342) ccw projected
  arc A166 (-128.0246, 103.9956) -> (-128.0089, 104.3948) centre (-148.5, 105) ccw projected
  arc A167 (-128.4867, 103.8371) -> (-128.0246, 103.9956) centre (-130.7166, 111.0894) ccw projected
  arc A168 (-128.867, 103.7329) -> (-128.4867, 103.8371) centre (-130.3699, 109.9618) ccw projected
  arc A169 (-129.1708, 103.669) -> (-128.867, 103.7329) centre (-130.1035, 108.8577) ccw projected
  arc A170 (-129.2005, 103.2909) -> (-129.1708, 103.669) centre (-148.5, 105) ccw projected
  arc A171 (-128.9105, 103.1803) -> (-129.2005, 103.2909) centre (-130.9335, 98.3119) ccw projected
  arc A172 (-128.5511, 103.0178) -> (-128.9105, 103.1803) centre (-131.3693, 97.2631) ccw projected
  arc A173 (-128.1196, 102.7889) -> (-128.5511, 103.0178) centre (-131.8881, 96.2037) ccw projected
  arc A174 (-128.1665, 102.3922) -> (-128.1196, 102.7889) centre (-148.5, 105) ccw projected
  arc A175 (-128.6396, 102.2705) -> (-128.1665, 102.3922) centre (-130.2936, 109.6753) ccw projected
  arc A176 (-129.027, 102.1964) -> (-128.6396, 102.2705) centre (-130.0365, 108.5241) ccw projected
  arc A177 (-129.3348, 102.1565) -> (-129.027, 102.1964) centre (-129.8575, 107.4025) ccw projected
  arc A178 (-129.3941, 101.7819) -> (-129.3348, 102.1565) centre (-148.5, 105) ccw projected
  arc A179 (-129.1137, 101.6489) -> (-129.3941, 101.7819) centre (-131.5124, 96.9543) ccw projected
  arc A180 (-128.7682, 101.4587) -> (-129.1137, 101.6489) centre (-132.0292, 95.9429) ccw projected
  arc A181 (-128.3559, 101.1967) -> (-128.7682, 101.4587) centre (-132.6295, 94.9274) ccw projected
  arc A182 (-128.4338, 100.8049) -> (-128.3559, 101.1967) centre (-148.5, 105) ccw projected
  arc A183 (-128.915, 100.7207) -> (-128.4338, 100.8049) centre (-129.983, 108.2324) ccw projected
  arc A184 (-129.307, 100.6772) -> (-128.915, 100.7207) centre (-129.8169, 107.0646) ccw projected
  arc A185 (-129.617, 100.6616) -> (-129.307, 100.6772) centre (-129.7265, 105.9324) ccw projected
  arc A186 (-129.7055, 100.2928) -> (-129.617, 100.6616) centre (-148.5, 105) ccw projected
  arc A187 (-129.4364, 100.1382) -> (-129.7055, 100.2928) centre (-132.196, 95.6463) ccw projected
  arc A188 (-129.1068, 99.9215) -> (-129.4364, 100.1382) centre (-132.7905, 94.6785) ccw projected
  arc A189 (-128.7164, 99.628) -> (-129.1068, 99.9215) centre (-133.4687, 93.7133) ccw projected
  arc A190 (-128.8248, 99.2435) -> (-128.7164, 99.628) centre (-148.5, 105) ccw projected
  arc A191 (-129.3111, 99.1972) -> (-128.8248, 99.2435) centre (-129.7864, 106.7696) ccw projected
  arc A192 (-129.7053, 99.1846) -> (-129.3111, 99.1972) centre (-129.7125, 105.5924) ccw projected
  arc A193 (-130.0156, 99.1934) -> (-129.7053, 99.1846) centre (-129.7112, 104.4566) ccw projected
  arc A194 (-130.1328, 98.8327) -> (-130.0156, 99.1934) centre (-148.5, 105) ccw projected
  arc A195 (-129.8766, 98.6575) -> (-130.1328, 98.8327) centre (-132.9801, 94.3959) ccw projected
  arc A196 (-129.5651, 98.4156) -> (-129.8766, 98.6575) centre (-133.6488, 93.4778) ccw projected
  arc A197 (-129.1989, 98.0923) -> (-129.5651, 98.4156) centre (-134.4006, 92.5688) ccw projected
  arc A198 (-129.3371, 97.7175) -> (-129.1989, 98.0923) centre (-148.5, 105) ccw projected
  arc A199 (-129.8255, 97.7096) -> (-129.3371, 97.7175) centre (-129.7053, 105.2959) ccw projected
  arc A200 (-130.2195, 97.728) -> (-129.8255, 97.7096) centre (-129.724, 104.1165) ccw projected
  arc A201 (-130.5281, 97.7611) -> (-130.2195, 97.728) centre (-129.8118, 102.9841) ccw projected
  arc A202 (-130.6733, 97.4107) -> (-130.5281, 97.7611) centre (-148.5, 105) ccw projected
  arc A203 (-130.4316, 97.2158) -> (-130.6733, 97.4107) centre (-133.86, 93.2109) ccw projected
  arc A204 (-130.14, 96.9503) -> (-130.4316, 97.2158) centre (-134.5986, 92.3481) ccw projected
  arc A205 (-129.8003, 96.5993) -> (-130.14, 96.9503) centre (-135.4194, 91.5009) ccw projected
  arc A206 (-129.9676, 96.2365) -> (-129.8003, 96.5993) centre (-148.5, 105) ccw projected
  arc A207 (-130.4551, 96.2669) -> (-129.9676, 96.2365) centre (-129.74, 103.8204) ccw projected
  arc A208 (-130.8464, 96.3161) -> (-130.4551, 96.2669) centre (-129.8512, 102.6461) ccw projected
  arc A209 (-131.1515, 96.3733) -> (-130.8464, 96.3161) centre (-130.0276, 101.524) ccw projected
  arc A210 (-131.3237, 96.0354) -> (-131.1515, 96.3733) centre (-148.5, 105) ccw projected
  arc A211 (-131.0981, 95.8222) -> (-131.3237, 96.0354) centre (-134.8301, 92.0986) ccw projected
  arc A212 (-130.8282, 95.5346) -> (-131.0981, 95.8222) centre (-135.6341, 91.2964) ccw projected
  arc A213 (-130.5171, 95.158) -> (-130.8282, 95.5346) centre (-136.5188, 90.5162) ccw projected
  arc A214 (-130.7123, 94.8095) -> (-130.5171, 95.158) centre (-148.5, 105) ccw projected
  arc A215 (-131.1959, 94.878) -> (-130.7123, 94.8095) centre (-129.8904, 102.3522) ccw projected
  arc A216 (-131.5822, 94.9578) -> (-131.1959, 94.878) centre (-130.0933, 101.1901) ccw projected
  arc A217 (-131.8818, 95.0388) -> (-131.5822, 94.9578) centre (-130.3572, 100.0854) ccw projected
  arc A218 (-132.08, 94.7154) -> (-131.8818, 95.0388) centre (-148.5, 105) ccw projected
  arc A219 (-131.8718, 94.4852) -> (-132.08, 94.7154) centre (-135.8844, 91.0659) ccw projected
  arc A220 (-131.6253, 94.1773) -> (-131.8718, 94.4852) centre (-136.7489, 90.3292) ccw projected
  arc A221 (-131.3447, 93.7774) -> (-131.6253, 94.1773) centre (-137.6922, 89.6208) ccw projected
  arc A222 (-131.5666, 93.4453) -> (-131.3447, 93.7774) centre (-148.5, 105) ccw projected
  arc A223 (-132.0434, 93.5515) -> (-131.5666, 93.4453) centre (-130.1555, 100.9002) ccw projected
  arc A224 (-132.4222, 93.6614) -> (-132.0434, 93.5515) centre (-130.449, 99.7577) ccw projected
  arc A225 (-132.7146, 93.7656) -> (-132.4222, 93.6614) centre (-130.7988, 98.6771) ccw projected
  arc A226 (-132.9375, 93.4588) -> (-132.7146, 93.7656) centre (-148.5, 105) ccw projected
  arc A227 (-132.748, 93.2129) -> (-132.9375, 93.4588) centre (-137.0166, 90.119) ccw projected
  arc A228 (-132.5265, 92.8866) -> (-132.748, 93.2129) centre (-137.9362, 89.4524) ccw projected
  arc A229 (-132.2781, 92.466) -> (-132.5265, 92.8866) centre (-138.9321, 88.8202) ccw projected
  arc A230 (-132.5254, 92.1523) -> (-132.2781, 92.466) centre (-148.5, 105) ccw projected
  arc A231 (-132.9924, 92.2957) -> (-132.5254, 92.1523) centre (-130.5337, 99.4736) ccw projected
  arc A232 (-133.3614, 92.4349) -> (-132.9924, 92.2957) centre (-130.9159, 98.3576) ccw projected
  arc A233 (-133.6447, 92.5617) -> (-133.3614, 92.4349) centre (-131.3494, 97.3078) ccw projected
  arc A234 (-133.891, 92.2734) -> (-133.6447, 92.5617) centre (-148.5, 105) ccw projected
  arc A235 (-133.7214, 92.0134) -> (-133.891, 92.2734) centre (-138.2195, 89.2639) ccw projected
  arc A236 (-133.5261, 91.6707) -> (-133.7214, 92.0134) centre (-139.1886, 88.6715) ccw projected
  arc A237 (-133.3115, 91.2319) -> (-133.5261, 91.6707) centre (-140.2311, 88.1194) ccw projected
  arc A238 (-133.5827, 90.9386) -> (-133.3115, 91.2319) centre (-148.5, 105) ccw projected
  arc A239 (-134.037, 91.1181) -> (-133.5827, 90.9386) centre (-131.0227, 98.081) ccw projected
  arc A240 (-134.3939, 91.2859) -> (-134.037, 91.1181) centre (-131.4913, 96.9985) ccw projected
  arc A241 (-134.6664, 91.4345) -> (-134.3939, 91.2859) centre (-132.0058, 95.9859) ccw projected
  arc A242 (-134.9345, 91.1664) -> (-134.6664, 91.4345) centre (-148.5, 105) ccw projected
  arc A243 (-134.7859, 90.8939) -> (-134.9345, 91.1664) centre (-139.4859, 88.5058) ccw projected
  arc A244 (-134.6181, 90.537) -> (-134.7859, 90.8939) centre (-140.4985, 87.9913) ccw projected
  arc A245 (-134.4386, 90.0827) -> (-134.6181, 90.537) centre (-141.581, 87.5227) ccw projected
  arc A246 (-134.7319, 89.8115) -> (-134.4386, 90.0827) centre (-148.5, 105) ccw projected
  arc A247 (-135.1707, 90.0261) -> (-134.7319, 89.8115) centre (-131.6194, 96.7311) ccw projected
  arc A248 (-135.5134, 90.2214) -> (-135.1707, 90.0261) centre (-132.1715, 95.6886) ccw projected
  arc A249 (-135.7734, 90.391) -> (-135.5134, 90.2214) centre (-132.7639, 94.7195) ccw projected
  arc A250 (-136.0617, 90.1447) -> (-135.7734, 90.391) centre (-148.5, 105) ccw projected
  arc A251 (-135.9349, 89.8614) -> (-136.0617, 90.1447) centre (-140.8078, 87.8494) ccw projected
  arc A252 (-135.7957, 89.4924) -> (-135.9349, 89.8614) centre (-141.8576, 87.4159) ccw projected
  arc A253 (-135.6523, 89.0254) -> (-135.7957, 89.4924) centre (-142.9736, 87.0337) ccw projected
  arc A254 (-135.966, 88.7781) -> (-135.6523, 89.0254) centre (-148.5, 105) ccw projected
  arc A255 (-136.3866, 89.0265) -> (-135.966, 88.7781) centre (-132.3202, 95.4321) ccw projected
  arc A256 (-136.7129, 89.248) -> (-136.3866, 89.0265) centre (-132.9524, 94.4362) ccw projected
  arc A257 (-136.9588, 89.4375) -> (-136.7129, 89.248) centre (-133.619, 93.5166) ccw projected
  arc A258 (-137.2656, 89.2146) -> (-136.9588, 89.4375) centre (-148.5, 105) ccw projected
  arc A259 (-137.1614, 88.9222) -> (-137.2656, 89.2146) centre (-142.1771, 87.2988) ccw projected
  arc A260 (-137.0515, 88.5434) -> (-137.1614, 88.9222) centre (-143.2577, 86.949) ccw projected
  arc A261 (-136.9453, 88.0666) -> (-137.0515, 88.5434) centre (-144.4002, 86.6555) ccw projected
  arc A262 (-137.2774, 87.8447) -> (-136.9453, 88.0666) centre (-148.5, 105) ccw projected
  arc A263 (-137.6773, 88.1253) -> (-137.2774, 87.8447) centre (-133.1208, 94.1922) ccw projected
  arc A264 (-137.9852, 88.3718) -> (-137.6773, 88.1253) centre (-133.8292, 93.2489) ccw projected
  arc A265 (-138.2154, 88.58) -> (-137.9852, 88.3718) centre (-134.5659, 92.3844) ccw projected
  arc A266 (-138.5388, 88.3818) -> (-138.2154, 88.58) centre (-148.5, 105) ccw projected
  arc A267 (-138.4578, 88.0822) -> (-138.5388, 88.3818) centre (-143.5854, 86.8572) ccw projected
  arc A268 (-138.378, 87.6959) -> (-138.4578, 88.0822) centre (-144.6901, 86.5933) ccw projected
  arc A269 (-138.3095, 87.2123) -> (-138.378, 87.6959) centre (-145.8522, 86.3904) ccw projected
  arc A270 (-138.658, 87.0171) -> (-138.3095, 87.2123) centre (-148.5, 105) ccw projected
  arc A271 (-139.0346, 87.3282) -> (-138.658, 87.0171) centre (-134.0162, 93.0188) ccw projected
  arc A272 (-139.3222, 87.5981) -> (-139.0346, 87.3282) centre (-134.7964, 92.1341) ccw projected
  arc A273 (-139.5354, 87.8237) -> (-139.3222, 87.5981) centre (-135.5986, 91.3301) ccw projected
  arc A274 (-139.8733, 87.6515) -> (-139.5354, 87.8237) centre (-148.5, 105) ccw projected
  arc A275 (-139.8161, 87.3464) -> (-139.8733, 87.6515) centre (-145.024, 86.5276) ccw projected
  arc A276 (-139.7669, 86.9551) -> (-139.8161, 87.3464) centre (-146.1461, 86.3512) ccw projected
  arc A277 (-139.7365, 86.4676) -> (-139.7669, 86.9551) centre (-147.3204, 86.24) ccw projected
  arc A278 (-140.0993, 86.3003) -> (-139.7365, 86.4676) centre (-148.5, 105) ccw projected
  arc A279 (-140.4503, 86.64) -> (-140.0993, 86.3003) centre (-135.0009, 91.9194) ccw projected
  arc A280 (-140.7158, 86.9316) -> (-140.4503, 86.64) centre (-135.8481, 91.0986) ccw projected
  arc A281 (-140.9107, 87.1733) -> (-140.7158, 86.9316) centre (-136.7109, 90.36) ccw projected
  arc A282 (-141.2611, 87.0281) -> (-140.9107, 87.1733) centre (-148.5, 105) ccw projected
  arc A283 (-141.228, 86.7195) -> (-141.2611, 87.0281) centre (-146.4841, 86.3118) ccw projected
  arc A284 (-141.2096, 86.3255) -> (-141.228, 86.7195) centre (-147.6165, 86.224) ccw projected
  arc A285 (-141.2175, 85.8371) -> (-141.2096, 86.3255) centre (-148.7959, 86.2053) ccw projected
  arc A286 (-141.5923, 85.6989) -> (-141.2175, 85.8371) centre (-148.5, 105) ccw projected
  arc A287 (-141.9156, 86.0651) -> (-141.5923, 85.6989) centre (-136.0688, 90.9006) ccw projected
  arc A288 (-142.1575, 86.3766) -> (-141.9156, 86.0651) centre (-136.9778, 90.1488) ccw projected
  arc A289 (-142.3327, 86.6328) -> (-142.1575, 86.3766) centre (-137.8959, 89.4801) ccw projected
  arc A290 (-142.6934, 86.5156) -> (-142.3327, 86.6328) centre (-148.5, 105) ccw projected
  arc A291 (-142.6846, 86.2053) -> (-142.6934, 86.5156) centre (-147.9566, 86.2112) ccw projected
  arc A292 (-142.6972, 85.8111) -> (-142.6846, 86.2053) centre (-149.0924, 86.2125) ccw projected
  arc A293 (-142.7435, 85.3248) -> (-142.6972, 85.8111) centre (-150.2696, 86.2864) ccw projected
  arc A294 (-143.128, 85.2164) -> (-142.7435, 85.3248) centre (-148.5, 105) ccw projected
  arc A295 (-143.4215, 85.6068) -> (-143.128, 85.2164) centre (-137.2133, 89.9687) ccw projected
  arc A296 (-143.6382, 85.9364) -> (-143.4215, 85.6068) centre (-138.1785, 89.2905) ccw projected
  arc A297 (-143.7928, 86.2055) -> (-143.6382, 85.9364) centre (-139.1463, 88.696) ccw projected
  arc A298 (-144.1616, 86.117) -> (-143.7928, 86.2055) centre (-148.5, 105) ccw projected
  arc A299 (-144.1772, 85.807) -> (-144.1616, 86.117) centre (-149.4324, 86.2265) ccw projected
  arc A300 (-144.2207, 85.415) -> (-144.1772, 85.807) centre (-150.5646, 86.3169) ccw projected
  arc A301 (-144.3049, 84.9338) -> (-144.2207, 85.415) centre (-151.7324, 86.483) ccw projected
  arc A302 (-144.6967, 84.8559) -> (-144.3049, 84.9338) centre (-148.5, 105) ccw projected
  arc A303 (-144.9587, 85.2682) -> (-144.6967, 84.8559) centre (-138.4274, 89.1295) ccw projected
  arc A304 (-145.1489, 85.6137) -> (-144.9587, 85.2682) centre (-139.4429, 88.5292) ccw projected
  arc A305 (-145.2819, 85.8941) -> (-145.1489, 85.6137) centre (-140.4543, 88.0124) ccw projected
  arc A306 (-145.6565, 85.8348) -> (-145.2819, 85.8941) centre (-148.5, 105) ccw projected
  arc A307 (-145.6964, 85.527) -> (-145.6565, 85.8348) centre (-150.9025, 86.3575) ccw projected
  arc A308 (-145.7705, 85.1396) -> (-145.6964, 85.527) centre (-152.0241, 86.5365) ccw projected
  arc A309 (-145.8922, 84.6665) -> (-145.7705, 85.1396) centre (-153.1753, 86.7936) ccw projected
  arc A310 (-146.2889, 84.6196) -> (-145.8922, 84.6665) centre (-148.5, 105) ccw projected
  arc A311 (-146.5178, 85.0511) -> (-146.2889, 84.6196) centre (-139.7037, 88.3881) ccw projected
  arc A312 (-146.6803, 85.4105) -> (-146.5178, 85.0511) centre (-140.7631, 87.8693) ccw projected
  arc A313 (-146.7909, 85.7005) -> (-146.6803, 85.4105) centre (-141.8119, 87.4335) ccw projected
  arc A314 (-147.169, 85.6708) -> (-146.7909, 85.7005) centre (-148.5, 105) ccw projected
  arc A315 (-147.2329, 85.367) -> (-147.169, 85.6708) centre (-152.3577, 86.6035) ccw projected
  arc A316 (-147.3371, 84.9867) -> (-147.2329, 85.367) centre (-153.4618, 86.8699) ccw projected
  arc A317 (-147.4956, 84.5246) -> (-147.3371, 84.9867) centre (-154.5894, 87.2166) ccw projected
  arc A318 (-147.8948, 84.5089) -> (-147.4956, 84.5246) centre (-148.5, 105) ccw projected
  arc A319 (-148.0891, 84.9571) -> (-147.8948, 84.5089) centre (-141.0342, 87.7492) ccw projected
  arc A320 (-148.2229, 85.3281) -> (-148.0891, 84.9571) centre (-142.131, 87.3151) ccw projected
  arc A321 (-148.3104, 85.6259) -> (-148.2229, 85.3281) centre (-143.2108, 86.9629) ccw projected
  arc A322 (-148.6896, 85.6259) -> (-148.3104, 85.6259) centre (-148.5, 105) ccw projected
  arc A323 (-148.7771, 85.3281) -> (-148.6896, 85.6259) centre (-153.7892, 86.9629) ccw projected
  arc A324 (-148.9109, 84.9571) -> (-148.7771, 85.3281) centre (-154.869, 87.3151) ccw projected
  arc A325 (-149.1052, 84.5089) -> (-148.9109, 84.9571) centre (-155.9658, 87.7492) ccw projected
  arc A326 (-149.5044, 84.5246) -> (-149.1052, 84.5089) centre (-148.5, 105) ccw projected
  arc A327 (-149.6629, 84.9867) -> (-149.5044, 84.5246) centre (-142.4106, 87.2166) ccw projected
  arc A328 (-149.7671, 85.367) -> (-149.6629, 84.9867) centre (-143.5382, 86.8699) ccw projected
  arc A329 (-149.831, 85.6708) -> (-149.7671, 85.367) centre (-144.6423, 86.6035) ccw projected
  arc A330 (-150.2091, 85.7005) -> (-149.831, 85.6708) centre (-148.5, 105) ccw projected
  arc A331 (-150.3197, 85.4105) -> (-150.2091, 85.7005) centre (-155.1881, 87.4335) ccw projected
  arc A332 (-150.4822, 85.0511) -> (-150.3197, 85.4105) centre (-156.2369, 87.8693) ccw projected
  arc A333 (-150.7111, 84.6196) -> (-150.4822, 85.0511) centre (-157.2963, 88.3881) ccw projected
  arc A334 (-151.1078, 84.6665) -> (-150.7111, 84.6196) centre (-148.5, 105) ccw projected
  arc A335 (-151.2295, 85.1396) -> (-151.1078, 84.6665) centre (-143.8247, 86.7936) ccw projected
  arc A336 (-151.3036, 85.527) -> (-151.2295, 85.1396) centre (-144.9759, 86.5365) ccw projected
  arc A337 (-151.3435, 85.8348) -> (-151.3036, 85.527) centre (-146.0975, 86.3575) ccw projected
  arc A338 (-151.7181, 85.8941) -> (-151.3435, 85.8348) centre (-148.5, 105) ccw projected
  arc A339 (-151.8511, 85.6137) -> (-151.7181, 85.8941) centre (-156.5457, 88.0124) ccw projected
  arc A340 (-152.0413, 85.2682) -> (-151.8511, 85.6137) centre (-157.5571, 88.5292) ccw projected
  arc A341 (-152.3033, 84.8559) -> (-152.0413, 85.2682) centre (-158.5726, 89.1295) ccw projected
  arc A342 (-152.6951, 84.9338) -> (-152.3033, 84.8559) centre (-148.5, 105) ccw projected
  arc A343 (-152.7793, 85.415) -> (-152.6951, 84.9338) centre (-145.2676, 86.483) ccw projected
  arc A344 (-152.8228, 85.807) -> (-152.7793, 85.415) centre (-146.4354, 86.3169) ccw projected
  arc A345 (-152.8384, 86.117) -> (-152.8228, 85.807) centre (-147.5676, 86.2265) ccw projected
  arc A346 (-153.2072, 86.2055) -> (-152.8384, 86.117) centre (-148.5, 105) ccw projected